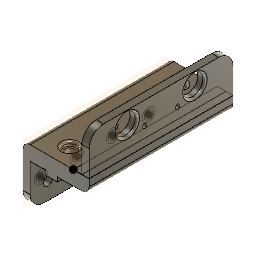
Extruder holder v4 (Autodesk Fusion 360 design; units mm, degrees)
Autodesk Fusion 360 part; units mm, degrees
sketch "Sketch1" plane through (0, 0, 0) normal (0, 0, 1) x (1, 0, 0)
  line L0 (0, 0) -> (30, 0)
  line L1 (30, 0) -> (30, 100)
  line L2 (30, 100) -> (0, 100)
  line L3 (0, 100) -> (0, 0)
  line L4 (15, 100) -> (15, 0) construction
  circle A0 centre (15, 12.6) radius 3.1
  circle A1 centre (15, 37.6) radius 3.1
  circle A2 centre (15, 62.6) radius 3.1
  circle A3 centre (15, 87.6) radius 3.1
  dimension "d1" = 100
  dimension "d2" = 30
  dimension "d3" = 6.2
  dimension "d6" = 1
  dimension "d7" = 25
  dimension "d11" = 12.6
  measures "d3" diameter of A0
extrude "Extrude1" add sketch "Sketch1" along normal blind 10
sketch "Sketch2" plane through (0, 0, 10) normal (0, 0, 1) x (-1, 0, 0)
  circle A0 centre (-15, -12.6) radius 3.1
  circle A1 centre (-15, -87.6) radius 3.1
  circle A2 centre (-15, -62.6) radius 3.1
  circle A3 centre (-15, -37.6) radius 3.1
  line L0 (0, -100) -> (0, 0)
  line L1 (0, 0) -> (-30, 0)
  line L2 (-30, 0) -> (-30, -100)
  line L3 (-30, -100) -> (0, -100)
  circle A4 centre (-15, -12.6) radius 4.5
  circle A5 centre (-15, -37.6) radius 4.5
  circle A6 centre (-15, -62.6) radius 4.5
  circle A7 centre (-15, -87.6) radius 4.5
  dimension "d17" = 9
  dimension "d20" = 0
  dimension "d21" = -25
  measures "d17" diameter of A4
extrude "Extrude2" cut sketch "Sketch2" against normal blind 3 contours A4 | A5 | A6 | A7
sketch "Sketch3" plane through (0, 0, 0) normal (0, 0, 1) x (1, 0, 0)
  line L0 (11, 0) -> (19, 0)
  line L1 (19, 0) -> (19, 100)
  line L2 (19, 100) -> (11, 100)
  line L3 (11, 100) -> (11, 0)
  line L4 (0, 0) -> (30, 0)
  line L5 (30, 100) -> (0, 100)
  line L6 (30, 0) -> (30, 100)
  dimension "d24" = 8
  dimension "d26" = 11
  measures "d24" distance of L1 L3
  measures "d26" distance of L1 L6
extrude "Extrude3" add sketch "Sketch3" against normal blind 3 contours L0 L1 L2 L3 L4 L5
extrude "Extrude4" cut sketch "Sketch1" against normal through all contours A0 | A1 | A2 | A3
sketch "Sketch4" plane through (0, 0, 10) normal (0, 0, 1) x (-1, 0, 0)
  circle A0 centre (-15, -37.6) radius 4.5
  circle A1 centre (-15, -62.6) radius 4.5
  circle A2 centre (-15, -12.6) radius 4.5
  circle A3 centre (-15, -87.6) radius 4.5
  line L0 (0, -100) -> (0, 0)
  line L1 (0, 0) -> (-30, 0)
  line L2 (-30, 0) -> (-30, -100)
  line L3 (-30, -100) -> (0, -100)
  line L4 (-30, 0) -> (-36, 0)
  line L5 (-36, 0) -> (-36, -100)
  line L6 (-36, -100) -> (-30, -100)
  line L7 (-30, -100) -> (-30, 0)
  line L8 (-36, 0) -> (-41, 0)
  line L9 (-41, 0) -> (-41, -100)
  line L10 (-41, -100) -> (-36, -100)
  line L11 (-36, -100) -> (-36, 0)
  dimension "d31" = 6
  dimension "d32" = 100
  dimension "d45" = 5
  dimension "d46" = 100
extrude "Extrude5" add sketch "Sketch4" against normal blind 10 contours L2 L4 L5 L6 L7 L11 | L5 L8 L9 L10 L11
extrude "Extrude6" add sketch "Sketch4" along normal blind 28 contours L5 L8 L9 L10 L11
sketch "Sketch5" plane through (41, 0, 0) normal (1, 0, 0) x (0, 1, 0)
  line L0 (0, 38) -> (0, 0)
  line L1 (0, 0) -> (100, 0)
  line L2 (100, 0) -> (100, 38)
  line L3 (100, 38) -> (0, 38)
  circle A0 centre (38.5, 22.5) radius 1.6
  line L4 (0, 10) -> (100, 10)
  circle A1 centre (61.5, 22.5) radius 1.6
  dimension "d47" = 3.2
  dimension "d49" = 12.5
  dimension "d50" = 3.2
  dimension "d51" = 23
  dimension "d52" = 12.5
  dimension "d53" = 38.5
  dimension "d54" = 38.5
  measures "d47" diameter of A0
  measures "d49" distance of L0.end L4
  measures "d50" diameter of A1
  measures "d52" distance of L4 L0.end
extrude "Extrude7" cut sketch "Sketch5" against normal through all contours A0 | A1
sketch "Sketch6" plane through (41, 0, 0) normal (1, 0, 0) x (0, 1, 0)
  circle A0 centre (38.5, 22.5) radius 1.6
  circle A1 centre (61.5, 22.5) radius 1.6
  line L0 (0, 38) -> (0, 0)
  line L1 (0, 0) -> (100, 0)
  line L2 (100, 0) -> (100, 38)
  line L3 (100, 38) -> (0, 38)
  circle A2 centre (73.5, 29) radius 7
  line L4 (50, 38) -> (50, 0) construction
  circle A3 centre (26.5, 29) radius 7
  dimension "d56" = 14
  dimension "d57" = 9
  dimension "d58" = 12
  measures "d56" diameter of A2
extrude "Extrude8" cut sketch "Sketch6" against normal through all contours A2 | A3
sketch "Sketch7" plane through (0, 0, 10) normal (0, 0, 1) x (-1, 0, 0)
  line L0 (0, 0) -> (5, 0)
  line L1 (5, 0) -> (5, -100)
  line L2 (5, -100) -> (0, -100)
  line L3 (0, -100) -> (0, 0)
  dimension "d60" = 100
  dimension "d61" = 5
  measures "d61" distance of L0.start
extrude "Extrude9" add sketch "Sketch7" against normal blind 40
sketch "Sketch8" plane through (-5, 0, 0) normal (-1, 0, 0) x (0, -1, 0)
  line L0 (0, 10) -> (-100, 10)
  line L1 (-100, 10) -> (-100, -30)
  line L2 (-100, -30) -> (0, -30)
  line L3 (0, -30) -> (0, 10)
  circle A0 centre (-87.4, -18.1) radius 3.1
  circle A1 centre (-87.4, -18.1) radius 4.5
  circle A2 centre (-62.4, -18.1) radius 3.1
  circle A3 centre (-62.4, -18.1) radius 4.5
  circle A4 centre (-37.4, -18.1) radius 3.1
  circle A5 centre (-37.4, -18.1) radius 4.5
  circle A6 centre (-12.4, -18.1) radius 3.1
  circle A7 centre (-12.4, -18.1) radius 4.5
  dimension "d64" = 6.2
  dimension "d65" = 9
  dimension "d66" = 11.9
  dimension "d69" = 25
  dimension "d70" = 0
  dimension "d71" = 12.6
  measures "d64" diameter of A0
  measures "d65" diameter of A1
  measures "d71" distance of L1
extrude "Extrude10" cut sketch "Sketch8" against normal through all contours A0 | A2 | A4 | A6
fillet "Fillet1" radius 10 4 edges at (38.5, 0, 38) (-2.5, 0, -30) (38.5, 100, 38) (-2.5, 100, -30)
fillet "Fillet2" radius 5 2 edges at (-5, 50, 10) (41, 50, 0)
fillet "Fillet3" radius 1.5 2 edges at (41, 19.9737, 31.5313) (41, 66.9737, 31.5313)
fillet "Fillet4" radius 1.5 4 edges at (19.1955, 85.9727, 10) (19.1955, 60.9727, 10) (19.1955, 35.9727, 10) (19.1955, 10.9727, 10)
equation "d1 = baseLenght"
equation "d2 = baseWidth"
equation "d7 = ( 100 / 4 ) * 1 mm"
equation "baseLenght = 100 mm"
equation "baseWidth = 30 mm"
equation "profileBoltDiameter = 6.2 mm"
equation "d11 = ( d1 / 4 ) - d3 * 2"
equation "baseThickness = 10 mm"
equation "d13 = baseThickness"
equation "profileBoltHeadDiameter = 9 mm"
equation "profileBoltHeadHeight = 3 mm"
equation "d17 = profileBoltHeadDiameter"
equation "d21 = -( baseLenght / 4 )"
equation "d22 = -profileBoltHeadHeight"
equation "d24 = profileGroove"
equation "profileGroove = 8 mm"
equation "d26 = ( baseWidth - profileGroove ) / 2"
equation "baseGrooveHeight = 3 mm"
equation "d28 = -baseGrooveHeight"
equation "d31 = prusaOffset"
equation "d32 = baseLenght"
equation "prusaOffset = 6 mm"
equation "frontWallThickness = 5 mm"
equation "d37 = -baseThickness"
equation "d42 = frontWallHeight"
equation "frontWallHeight = 28 mm"
equation "d45 = frontWallThickness"
equation "d46 = baseLenght"
equation "d47 = connectionBolt"
equation "connectionBolt = 3.2 mm"
equation "d50 = d47"
equation "d52 = d49"
equation "d53 = ( baseLenght - d51 ) / 2"
equation "d60 = baseLenght"
equation "d61 = frontWallThickness"
equation "d62 = -baseWidth - baseThickness"
equation "d64 = profileBoltDiameter"
equation "d65 = profileBoltHeadDiameter"
equation "d66 = ( baseWidth - profileBoltDiameter ) / 2"
equation "d69 = baseLenght / 4"
equation "d71 = baseLenght / 4 - profileBoltDiameter * 2"
